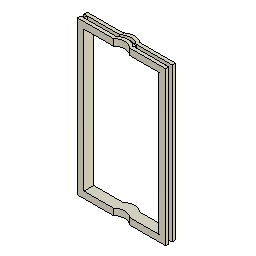
BATERIA_BARCO v2 (Autodesk Fusion 360 design; units mm, degrees)
Autodesk Fusion 360 part; units mm, degrees
sketch "Esboço1" plane through (0, 0, 0) normal (0, 0, 1) x (1, 0, 0)
  line L0 (54, 0) -> (52, 0)
  line L1 (52, 0) -> (52, 2)
  line L2 (2, 2) -> (2, 0)
  line L3 (2, 2) -> (0, 2)
  line L4 (0, 2) -> (0, 4)
  line L5 (54, 4) -> (54, 2)
  line L6 (54, 2) -> (52, 2)
  line L7 (54, 0) -> (54, -2)
  line L8 (0, -2) -> (0, 0)
  arc A0 (31.9959, 2) -> (21.9959, 2) centre (26.9959, -3.25) ccw
  arc A1 (32, 4) -> (22, 4) centre (27, -1.25) ccw
  line L9 (0, 4) -> (22, 4)
  line L10 (32, 4) -> (54, 4)
  arc A2 (32, 0) -> (22, 0) centre (27, -5.25) ccw
  line L11 (52, 2) -> (31.9959, 2)
  line L12 (21.9959, 2) -> (2, 2)
  arc A3 (32, -2) -> (22, -2) centre (27, -7.25) ccw
  line L13 (54, -2) -> (32, -2)
  line L14 (22, -2) -> (0, -2)
  line L15 (0, 0) -> (22, 0)
  line L16 (32, 0) -> (54, 0)
  dimension "d1" = 54
  dimension "d2" = 50
  constraint coincident L8.end L15.start
  constraint horizontal L15
  constraint coincident L0.end L15
  constraint perpendicular L1 L15
  constraint perpendicular L1 L11
  constraint coincident L2.end L15
  constraint perpendicular L2 L15
  constraint perpendicular L2 L3
  constraint perpendicular L3 L4
  constraint perpendicular L4 L9
  constraint perpendicular L5 L9
  constraint perpendicular L1 L6
  constraint perpendicular L0 L7
  constraint perpendicular L7 L13
  constraint perpendicular L8 L15
  constraint coincident A0.end L11
  constraint tangent A0 L9
  constraint collinear L9 L10
  constraint coincident A2.start L15
  constraint collinear L11 L12
  constraint coincident A3.end L13
  constraint collinear L13 L14
  constraint collinear L15 L16
  measures "d1" distance of L8.end L0.start
  measures "d2" distance of L1.end L2.start
extrude "Extrusão1" add sketch "Esboço1" along normal blind 94
sketch "Esboço2" plane through (0, 0, 94) normal (0, 0, 1) x (-1, 0, 0)
  arc A0 (-32, -4) -> (-22, -4) centre (-27, 1.25) ccw
  line L0 (-22, -4) -> (0, -4)
  line L1 (0, -4) -> (0, -2)
  line L2 (0, -2) -> (-2, -2)
  line L3 (-2, -2) -> (-2, 0)
  line L4 (-2, 0) -> (0, 0)
  line L5 (0, 0) -> (0, 2)
  line L6 (0, 2) -> (-22, 2)
  arc A1 (-32, 2) -> (-22, 2) centre (-27, 7.25) ccw
  line L7 (-32, 2) -> (-54, 2)
  line L8 (-54, 2) -> (-54, 0)
  line L9 (-54, 0) -> (-52, 0)
  line L10 (-52, 0) -> (-52, -2)
  line L11 (-52, -2) -> (-54, -2)
  line L12 (-54, -2) -> (-54, -4)
  line L13 (-54, -4) -> (-32, -4)
  line L14 (-52.0041, -2) -> (-32, -2)
  arc A2 (-32, -2) -> (-22, -2) centre (-27, 3.25) ccw
  line L15 (-22, -2) -> (-2.0041, -2)
  line L16 (-52.0041, -2) -> (-32, -2)
  arc A3 (-32, -2) -> (-22, -2) centre (-27, 3.25) ccw
  line L17 (-22, -2) -> (-2.0041, -2)
  line L18 (-52.0041, 0) -> (-32, 0)
  arc A4 (-32, 0) -> (-22, 0) centre (-27, 5.25) ccw
  line L19 (-22, 0) -> (-2.0041, 0)
  line L20 (-52.0041, 0) -> (-52.0041, -2)
  line L21 (-2, 0) -> (-2.0041, -2)
  line L22 (-2, 0) -> (-22, 0)
  line L23 (-32, 0) -> (-52, 0)
  dimension "d10" = 50
  dimension "d11" = 50
  dimension "d12" = 50
  constraint coincident A2.end L14
  constraint collinear L14 L15
  constraint coincident A2.end L16
  constraint collinear L16 L17
  constraint coincident A4.end L18
  constraint collinear L18 L19
  constraint perpendicular L14 L20
  constraint coincident L3.end L4.start
  constraint coincident L9.end L10.start
  measures "d10" distance of L15.end L14.start
  measures "d11" distance of L15.end L14.start
  measures "d12" distance of L18.start L19.end
extrude "Extrusão2" add sketch "Esboço1" along normal blind 12 contours L1 L2 A0 A2 L11 L12 L15 L16
extrude "Extrusão4" cut sketch "Esboço2" against normal blind 2 contours L10 L14 A2 L15 L16 A3 L17 L18 A4 L19 L21 L22 L23
extrude "Extrusão6" cut sketch "Esboço1" along normal blind 2 contours L1 L2 A0 A2 L11 L12 L15 L16
sketch "Esboço3" plane through (0, 4, 0) normal (0, 1, 0) x (-1, 0, 0)
  line L0 (-22, 0) -> (0, 0)
  line L1 (0, 0) -> (0, 94)
  line L2 (0, 94) -> (-22, 94)
  line L3 (-22, 94) -> (-22, 0)
ref_plane "Plano de trabalho1" through (11, 4, 47) normal (0, 1, 0) x (-1, 0, 0)
sketch "Esboço4" plane through (11, 4, 47) normal (0, 1, 0) x (-1, 0, 0)
  line L0 (-40, -47) -> (-40, -45)
  line L1 (-43, -45) -> (-41, -45)
  line L2 (-39, 43) -> (7, 43)
  line L3 (7, -43) -> (7, 43)
  line L4 (-39, -43) -> (7, -43)
  line L5 (-39, -43) -> (-39, 43)
  dimension "d26" = 2
  constraint vertical L0
  constraint horizontal L1
  measures "d26" distance of L0.start L0.end
extrude "Extrusão7" cut sketch "Esboço4" against normal blind 15
sketch "Esboço5" plane through (0, 4, 0) normal (0, -1, 0) x (1, 0, 0)
  line L0 (32, 4) -> (32, 90)
  line L1 (32, 90) -> (22, 90)
  line L2 (22, 90) -> (22, 4)
  line L3 (22, 4) -> (32, 4)
  line L4 (22, 4) -> (22, 6)
  line L5 (22, 6) -> (32, 6)
  line L6 (32, 90) -> (32, 88)
  line L7 (32, 88) -> (22, 88)
  line L8 (22, 88) -> (22, 6)
  line L9 (32, 6) -> (32, 88)
  dimension "d31" = 2
  dimension "d32" = 2
  constraint coincident L2.end L3.start
  constraint perpendicular L3 L4
  constraint coincident L0 L5.end
  constraint perpendicular L0 L5
  constraint coincident L0.end L1.start
  constraint perpendicular L1 L6
  constraint coincident L2 L7.end
  constraint perpendicular L2 L7
  measures "d31" distance of L2.end L4.end
  measures "d32" distance of L0.end L6.end
extrude "Extrusão8" cut sketch "Esboço5" against normal blind 25 contours L0 L2 L5 L7 L8 L9
move_face "Deslocar faces1" offset 1 1 faces at (28.6667, 4, 4.6667)
extrude "Extrusão9" cut 1 faces at (28.9579, 3, 5.3333) along direction (0, 1, 0) blind 8
extrude "Extrusão10" cut 1 faces at (25.3333, 4, 88.6667) along direction (0, 1, 0) blind 9
extrude "Extrusão5" [suppressed]
extrude "Extrusão3" [suppressed]
